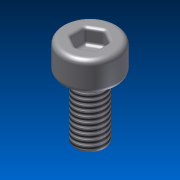
# Autodesk Inventor part: Cap(M3-6)
Saved by Autodesk Inventor 2013 (Build 170138000, 138)
## iProperties
Created: 2014-02-07
Material: 一般
Document SubType Name: Modeling
Designer: andou
Density: 1 g/cm^3
Mass: 0.103642 g
Surface Area: 1.57529 cm^2
Volume: 0.103642 cm^3
Author: andou
Title: Cap(M3-6)
Autodesk Inventor part; units mm, degrees
ref_plane "YZ Plane" through (0, 0, 0) normal (1, 0, 0) x (0, 1, 0)
ref_plane "XZ Plane" through (0, 0, 0) normal (0, 1, 0) x (-1, 0, 0)
ref_plane "XY Plane" through (0, 0, 0) normal (0, 0, 1) x (1, 0, 0)
sketch "スケッチ1" plane through (0, 0, 0) normal (0, 0, 1) x (1, 0, 0)
  circle A0 centre (0, 0) radius 2.75
  dimension "d0" = 5.5
  constraints: 1 centre point, 1 coincident
  measures "d0" diameter of A0
extrude "押し出し1" add sketch "スケッチ1" along normal blind 3
sketch "スケッチ2" plane through (0, 0, 0) normal (0, 0, -1) x (-1, 0, 0)
  circle A0 centre (0, 0) radius 2.75 projected
  circle A1 centre (0, 0) radius 1.5
  dimension "d3" = 3
  constraints: 1 centre point, 1 coincident
  measures "d3" diameter of A1
extrude "押し出し2" add sketch "スケッチ2" along normal blind 6 contours A1
sketch "スケッチ3" plane through (0, 0, 3) normal (0, 0, 1) x (1, 0, 0)
  circle A0 centre (0, 0) radius 2.75 projected
  line L0 (0, 1.4434) -> (1.25, 0.7217)
  line L1 (1.25, 0.7217) -> (1.25, -0.7217)
  line L2 (1.25, -0.7217) -> (0, -1.4434)
  line L3 (0, -1.4434) -> (-1.25, -0.7217)
  line L4 (-1.25, -0.7217) -> (-1.25, 0.7217)
  line L5 (-1.25, 0.7217) -> (0, 1.4434)
  dimension "d6" = 1.25
  constraints: 12 end point, 1 coincident, 13 other
  measures "d6" distance from line of point (0, 0) L0
extrude "押し出し3" cut sketch "スケッチ3" against normal blind 1.5 contours L0 L1 L2 L3 L4 L5
fillet "フィレット1" radius 0.5 2 edges at (-2.75, 0, 3) (-2.75, 0, 0)
fillet "フィレット2" radius 0.3 19 edges at (-0.625, 1.0825, 3) (-1.25, 0, 3) (-0.625, -1.0825, 3) (0.625, -1.0825, 3) (1.25, 0, 3) (0.625, 1.0825, 3) (-0.625, 1.0825, 1.5) (0.625, 1.0825, 1.5) (0, 1.4434, 2.25) (-1.25, 0.7217, 2.25) (-0.625, -1.0825, 1.5) (-1.25, -0.7217, 2.25) (-1.25, 0, 1.5) (1.25, 0, 1.5) (1.25, 0.7217, 2.25) (1.25, -0.7217, 2.25) (0.625, -1.0825, 1.5) (0, -1.4434, 2.25) (1.5, 0, -6)
thread "ねじ2" size "M3x0.5" class "6g" standard "ANSI Metric M Profile" full length
